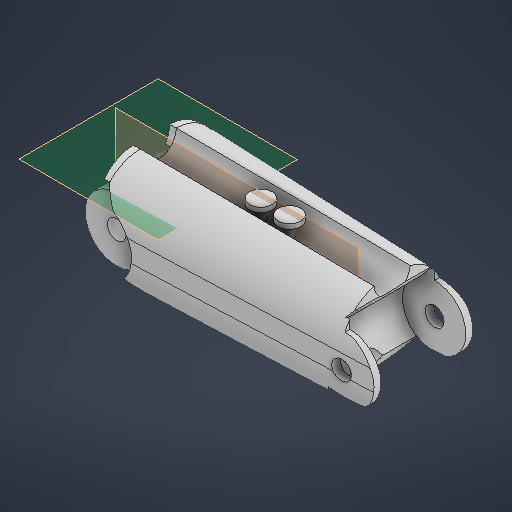
# Autodesk Inventor part: falange2_anular_V13
Saved by Autodesk Inventor 2026.1 (Build 301233020, 233B)
## iProperties
Created: 2026-01-14
Part Number: falange2_anular_V13
Material: Generic
Document SubType Name: Modeling
Designer: user
Density: 1 g/cm^3
Appearance: Default
Author: user
Autodesk Inventor part; units mm, degrees
ref_plane "YZ Plane" through (0, 0, 0) normal (1, 0, 0) x (0, 1, 0)
ref_plane "XY Plane" through (0, 0, 0) normal (0, 0, 1) x (1, 0, 0)
sketch "Sketch1" plane through (0, 0, 0) normal (0, 0, 1) x (1, 0, 0)
  line L0 (5.2681, -7.5236) -> (31.7319, -7.5236)
  circle A0 centre (0, 0) radius 1.5
  line L1 (0, 5) -> (0, 9.2)
  circle A1 centre (37, 0) radius 1.5
  arc A2 (34.1751, -4.0343) -> (37, 4.925) centre (37, 0) ccw
  line L2 (37, 4.925) -> (37, 9.075)
  line L3 (37, 9.075) -> (0, 9.2)
  arc A3 (0, 5) -> (2.8679, -4.0958) centre (0, 0) ccw
  line L4 (2.8679, -4.0958) -> (5.2681, -7.5236)
  line L5 (34.1751, -4.0343) -> (31.7319, -7.5236)
  dimension "d13" = 3
  dimension "d36" = 3
  dimension "d37" = 9.85
  dimension "d65" = 0
  dimension "d66" = 37
  dimension "d67" = 4.15
  dimension "d73" = 10
  dimension "d112" = 4.2
  dimension "d144" = 55
  dimension "d172" = 4.2596
  dimension "d173" = 4.1846
  dimension "d174" = 55
  constraints: 12 end point, 4 centre point, 4 point on circle, 3 coincident, 2 vertical, 1 parallel
  measures "d13" diameter of A0
  measures "d36" diameter of A1
  measures "d37" diameter of A2
  measures "d65" vertical distance of point (0, 0) A1.centre
  measures "d66" distance of A1.centre point (0, 0)
  measures "d67" distance of L2.start L2.end
  measures "d73" diameter of A3
  measures "d112" distance of L1.start L1.end
  measures "d144" angle of L0 L4
  measures "d172" distance of L5.start L0.end
  measures "d173" distance of L4.start L0.start
  measures "d174" angle of L0 L5
extrude "Extrusion1" add sketch "Sketch1" along normal mid plane 23
sketch "Sketch4" plane through (0, 9.2, -11.5) normal (-1, 0, 0) x (0, 0, 1)
  circle A0 centre (11.5, -13.8108) radius 1.5
  point P0 (11.5, -9.2)
  dimension "d23" = 3
  constraints: 1 centre point
  measures "d23" diameter of A0
extrude "Extrusion4" cut sketch "Sketch4" against normal through all
sketch "Sketch7" plane through (0, 0, 0) normal (0, 0, 1) x (1, 0, 0)
  circle A0 centre (37, 0) radius 5.075
  circle A1 centre (37, 0) radius 1.5 projected
  point P0 (0, 0)
  dimension "d116" = 10.15
  dimension "d178" = 0
  constraints: 1 centre point, 1 coincident
  measures "d116" diameter of A0
  measures "d178" distance of A1.centre point (37, 0)
extrude "Extrusion6" cut sketch "Sketch7" along normal mid plane 13.41 contours A0 | A1
ref_plane "Work Plane4" through (0, 0, 0) normal (0, 0, 1) x (1, 0, 0)
sketch "Sketch14" plane through (0, 0, 0) normal (0, 0, 1) x (1, 0, 0)
  circle A0 centre (0, 0) radius 5
  dimension "d80" = 10
  constraints: 1 centre point, 1 coincident
  measures "d80" diameter of A0
extrude "Extrusion12" cut sketch "Sketch14" along normal mid plane 3.825
sketch "Sketch39" plane through (5.2681, -7.5236, 11.5) normal (0, -1, 0) x (1, 0, 0)
  line L0 (-5.2681, -11.5) -> (20.8531, -11.5)
  line L1 (-5.2681, -2) -> (-27.6718, -2)
  line L2 (-27.6718, -2) -> (-27.6718, -11.5)
  line L3 (-27.6718, -11.5) -> (-5.2681, -11.5)
  line L4 (36.6569, 0.1344) -> (36.6569, -11.5)
  line L5 (36.6569, -11.5) -> (20.8531, -11.5)
  line L6 (-27.6718, -21) -> (-27.6718, -11.5)
  line L7 (-5.2681, -21) -> (-27.6718, -21)
  line L8 (36.6569, -23.1344) -> (36.6569, -11.5)
  line L9 (31.7319, 0) -> (-5.2681, 0) projected
  line L10 (-5.2681, -23) -> (31.7319, -23) projected
  line L11 (-3.7681, -23) -> (-6.7681, -23) projected
  line L12 (-5.2681, -2) -> (-5.2681, 0)
  line L13 (-5.2681, -21) -> (-5.2681, -23)
  line L14 (-40.5375, -11.5) -> (49.5226, -11.5) projected
  line L15 (31.7319, -4.795) -> (31.7319, -18.205) projected
  line L16 (31.7319, -23) -> (31.7319, 0) projected
  line L17 (31.7319, -11.5) -> (31.7319, -3.5)
  line L18 (-5.2681, -21) -> (36.6569, -19.3003)
  line L19 (-5.2681, -2) -> (36.6569, -3.6997)
  line L20 (36.6569, -4.795) -> (36.6569, 0) projected
  point P0 (-4.1469, -11.0242)
  point P1 (-3.1099, -9.8168)
  point P2 (20.8531, -20)
  point P3 (31.7319, -19.5)
  dimension "d161" = 9.5
  dimension "d162" = -23.963
  dimension "d168" = 0
  dimension "d169" = 8
  dimension "d180" = 0
  constraints: 28 end point, 5 symmetric about line, 3 perpendicular, 3 point on line, 2 horizontal, 2 vertical, 1 collinear, 1 midpoint, 1 parallel
  measures "d161" distance of L0.start L1.start
  measures "d162" horizontal distance of point (-3.11, -9.817) L0.end
  measures "d168" distance between parallel lines of L14 L3
  measures "d169" distance of L17.start L17.end
  measures "d180" distance between parallel lines of L20 L4
extrude "Extrusion24" cut sketch "Sketch39" against normal blind 24 contours L3 L2 L1 L19 L16 L15 L5 L0 | L0 L5 L15 L16 L18 L7 L6 L3 | L15 L16 L19 L4 L5 | L5 L8 L18 L16 L15 keep common part
fillet "Fillet5" radius 6.7625 2 edges at (18.5, -7.5236, -8.75) (18.5, -7.5236, 8.75)
fillet "Fillet6" radius 6.7625 2 edges at (18.5, 9.1375, 8.75) (18.5, 9.1375, -8.75)
sketch "Sketch12" plane through (0, 0, 11.5) normal (0, 0, 1) x (1, 0, 0)
  circle A0 centre (0, 0) radius 1.5 projected
  circle A1 centre (0, 0) radius 5.075
  dimension "d74" = 10.15
  constraints: 1 centre point, 1 coincident
  measures "d74" diameter of A1
extrude "Extrusion10" cut sketch "Sketch12" against normal blind 4.945
sketch "Sketch13" plane through (0, 0, -11.5) normal (0, 0, -1) x (-1, 0, 0)
  circle A0 centre (0, 0) radius 5.075
  dimension "d77" = 10.15
  constraints: 1 centre point
  measures "d77" diameter of A0
extrude "Extrusion11" cut sketch "Sketch13" against normal blind 4.945
sketch "Sketch16" plane through (0, 0, 0) normal (0, 0, 1) x (1, 0, 0)
  circle A0 centre (0, 0) radius 1.5 projected
  line L0 (-1.9036, 2.4472) -> (1.1675, 2.8722)
  line L1 (1.1675, 2.8722) -> (3.0711, 0.425)
  line L2 (3.0711, 0.425) -> (1.9036, -2.4472)
  line L3 (1.9036, -2.4472) -> (-1.1675, -2.8722)
  line L4 (-1.1675, -2.8722) -> (-3.0711, -0.425)
  line L5 (-3.0711, -0.425) -> (-1.9036, 2.4472)
  dimension "d83" = 5.37
  constraints: 12 end point, 1 coincident, 13 other
  measures "d83" distance between parallel lines of L3 L0
extrude "Extrusion13" cut sketch "Sketch16" along normal mid plane 8.085 contours A0 | L0 L1 L2 L3 L4 L5
ref_plane "Work Plane1" through (0, 9.2, -11.5) normal (0, 1, 0) x (-1, 0, 0)
sketch "Sketch27" plane through (37, 4.925, -11.5) normal (1, 0, 0) x (0, 0, -1)
  line L0 (0, 4.15) -> (-23, 4.15) projected
  circle A0 centre (-11.5, 4.15) radius 2.8604
  point P0 (-11.5, -4.925)
  dimension "d117" = 5.7208
  constraints: 1 centre point, 1 midpoint
  measures "d117" diameter of A0
sketch "Sketch28" plane through (0, 9.2, 11.5) normal (0.0033784, 0.9999943, 0) x (0.9999943, -0.0033784, 0)
  line L0 (37.0002, 23) -> (37.0002, 0) projected
  line L1 (37.0002, 11.5) -> (-0.9689, 11.5)
  point P0 (0.0311, 11.5)
  dimension "d175" = 1
  constraints: 2 end point, 1 horizontal, 1 midpoint
  measures "d175" distance of point (0.031, 11.5) L1.end
sweep "Sweep1" cut profiles "Sketch27" path "Sketch28" path curves L1
ref_plane "Work Plane2" through (0, 6.3396, 0) normal (-0.0033784, -0.9999943, 0) x (0.9999943, -0.0033784, 0)
sketch "Sketch30" plane through (0, 6.3396, 0) normal (-0.0033784, -0.9999943, 0) x (0.9999943, -0.0033784, 0)
  line L0 (36.9905, 0) -> (20.7505, 0)
  circle A0 centre (20.7505, 0) radius 0.7321
  ellipse E0 centre (36.9905, 0) end of major axis (36.9905, 2.8604) minor radius 0.0097 (36.9912, -2.8536) -> (36.9912, 2.8536) ccw projected
  point P0 (0.0214, 0)
  point P1 (59.9942, -2.8604)
  point P2 (59.9942, 2.8604)
  dimension "d122" = 16.24
  dimension "d123" = 1.4642
  dimension "d177" = 0
  constraints: 2 end point, 1 centre point, 1 coincident, 1 horizontal, 1 other
  measures "d122" distance of L0.start L0.end
  measures "d123" diameter of A0
  measures "d177" distance of point (36.991, 0) L0.start
extrude "Extrusion19" add sketch "Sketch30" against normal blind 2.1075
sketch "Sketch31" plane through (20.7575, 8.377, 0) normal (0.0033784, 0.9999943, 0) x (0.9999943, -0.0033784, 0)
  circle A0 centre (0, 0) radius 0.7321 projected
  circle A1 centre (0, 0) radius 1.774
  point P0 (-20.7291, 0)
  dimension "d126" = 3.548
  constraints: 1 centre point, 1 coincident
  measures "d126" diameter of A1
extrude "Extrusion20" add sketch "Sketch31" along normal up to surface (0.7529 mm away) contours A0 | A1
sketch "Sketch34" plane through (0, 6.3396, 0) normal (-0.0033784, -0.9999943, 0) x (0.9999943, -0.0033784, 0)
  ellipse E0 centre (36.9905, 0) end of major axis (36.9905, 2.8604) minor radius 0.0097 (36.9912, -2.8536) -> (36.9912, 2.8536) ccw projected
  ellipse E1 centre (-0.0097, 0) end of major axis (-0.0097, -2.8604) minor radius 0.0097 (-0.0097, -2.8604) -> (-0.0097, 2.8604) ccw projected
  line L0 (-0.0097, 0) -> (16.2303, 0)
  circle A0 centre (16.2303, 0) radius 0.7321
  point P0 (0.0214, 0)
  point P1 (59.9942, -2.8604)
  point P2 (59.9942, 2.8604)
  point P3 (-0.006, 2.8604)
  point P4 (-0.006, -2.8604)
  dimension "d130" = 16.24
  dimension "d131" = 1.4642
  constraints: 2 end point, 1 centre point, 1 coincident, 1 horizontal, 2 other
  measures "d130" distance of L0.start L0.end
  measures "d131" diameter of A0
extrude "Extrusion21" add sketch "Sketch34" against normal blind 2.1075
sketch "Sketch35" plane through (16.2374, 8.3923, 0) normal (0.0033784, 0.9999943, 0) x (0.9999943, -0.0033784, 0)
  circle A0 centre (0, 0) radius 0.7321 projected
  circle A1 centre (0, 0) radius 1.774
  point P0 (-16.2089, 0)
  dimension "d134" = 3.548
  constraints: 1 centre point, 1 coincident
  measures "d134" diameter of A1
extrude "Extrusion22" add sketch "Sketch35" along normal up to surface (0.7529 mm away) contours A0 | A1
chamfer "Chamfer1" distance 2 angle 45 1 edges at (37, 5.075, 0)
chamfer "Chamfer2" distance 2 angle 45 2 edges at (0, 5.075, -7.7597) (0, 5.075, 7.7597)
sketch "Sketch36" plane through (0, 5, -6.555) normal (-1, 0, 0) x (0, 0, 1)
  arc A0 (3.6946, 4.1988) -> (9.4154, 4.1988) centre (6.555, 4.2) ccw projected
  arc A1 (8.4697, 2.075) -> (9.4154, 4.2) centre (6.555, 4.2) ccw
  arc A2 (6.555, 1.3396) -> (9.4154, 4.2) centre (6.555, 4.2) ccw
  line L0 (6.555, 5.0268) -> (6.555, -0.0494)
  arc A3 (3.6946, 4.2) -> (4.6403, 2.075) centre (6.555, 4.2) ccw
  line L1 (0, -10) -> (0, 0) projected
  line L2 (3.9417, -5) -> (10.0382, -5)
  ellipse E0 centre (3.8231, -2.5625) end of major axis (-2.9217, -2.0005) minor radius 6.7625 (3.6946, 4.1988) -> (-1.1035, 2.075) ccw projected
  ellipse E1 centre (9.2869, -2.5625) end of major axis (16.0317, -2.0005) minor radius 6.7625 (14.2135, 2.075) -> (9.4154, 4.1988) ccw projected
  line L3 (0, 2.075) -> (-1.1035, 2.075) projected
  line L4 (0, 2.075) -> (0, 0) projected
  line L5 (0, 2.075) -> (4.6403, 2.075)
  line L6 (13.11, 2.075) -> (8.4697, 2.075)
  line L7 (14.2135, 2.075) -> (13.11, 2.075) projected
  point P0 (6.555, -5)
  point P1 (8.4697, 2.075)
  point P2 (4.6403, 2.075)
  point P3 (3.6946, 4.1988)
  point P4 (4.6403, 2.075)
  point P5 (-4.945, 2.075)
  point P6 (18.055, 2.075)
  point P7 (3.6946, 4.1989)
  point P8 (9.4154, 4.1989)
  constraints: 8 end point, 7 point on circle, 3 centre point, 2 coincident, 2 concentric, 2 symmetric about line, 1 collinear, 1 horizontal, 1 vertical, 3 other
revolve "Revolution1" add sketch "Sketch36" angle 7 about axis through (0, 0, -2.6133) along (0, 0, 1)
equation "\"d13\" = diametroDentroUnion"
equation "\"d36\" = diametroDentroUnion"
equation "\"d73\" = diametroFueraUnion"
equation "\"d80\" = diametroFueraUnion"
equation "\"d16\" = 135deg"
equation "\"d26\" = 135deg"
equation "\"d27\" = 135deg"
equation "\"d30\" = 135deg"
equation "\"d34\" = 23"
equation "\"d35\" = 0"
equation "\"d40\" = 135deg"
equation "\"d41\" = 10.639"
equation "\"d42\" = 11.8875"
equation "\"d43\" = 0"
equation "\"diametroDentroUnion\" = 3"
equation "\"diametroFueraUnion\" = 10"
equation "\"d45\" = 15"
equation "\"d39\" = diametroDentroUnion"
equation "\"tolerancia\" = 0.15"
body "Solid1"
